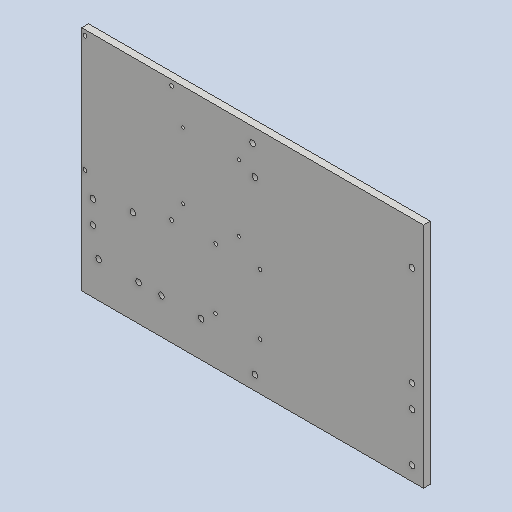
# Autodesk Inventor part: BackPlate
Saved by Autodesk Inventor 2023 (Build 270158000, 158)
## iProperties
Created: 2022-08-30
Part Number: BackPlate
Material: Generic
Document SubType Name: Modeling
Designer: Nathann
Density: 1 g/cm^3
Appearance: Default
Author: Nathann
Autodesk Inventor part; units mm, degrees
ref_plane "YZ Plane" through (0, 0, 0) normal (1, 0, 0) x (0, 1, 0)
ref_plane "XZ Plane" through (0, 0, 0) normal (0, 1, 0) x (-1, 0, 0)
ref_plane "XY Plane" through (0, 0, 0) normal (0, 0, 1) x (1, 0, 0)
sketch "Sketch1" plane through (0, 0, 0) normal (0, 1, 0) x (-1, 0, 0)
  line L0 (-150, -100) -> (150, -100)
  line L1 (150, -100) -> (150, 100)
  line L2 (150, 100) -> (-150, 100)
  line L3 (-150, 100) -> (-150, -100)
  line L4 (-150, -100) -> (150, 100) construction
  line L5 (150, -100) -> (-150, 100) construction
  point P0 (0, 0)
  dimension "d2" = 200
  dimension "d3" = 300
  constraints: 12 end point, 2 midpoint, 2 parallel, 1 horizontal, 1 perpendicular
  measures "d2" distance of L2.end L0.start
  measures "d3" distance of L0.start L0.end
extrude "Extrusion1" add sketch "Sketch1" along normal blind 6
sketch "Sketch2" plane through (0, 0, 0) normal (0, -1, 0) x (1, 0, 0)
  circle A0 centre (-11.9893, 68.6126) radius 1.35 projected
  circle A1 centre (-32.5352, -58.3765) radius 1.6 projected
  circle A2 centre (-32.4109, -5.3766) radius 1.6 projected
  circle A3 centre (6.589, -5.468) radius 1.6 projected
  circle A4 centre (-61.0635, 10.6754) radius 1.35 projected
  circle A5 centre (6.4647, -58.4679) radius 1.6 projected
  circle A6 centre (-12.0636, 10.6126) radius 1.35 projected
  circle A7 centre (-71.0314, 95.3283) radius 1.75 projected
  circle A8 centre (-147.0245, -6.6768) radius 1.75 projected
  circle A9 centre (-71.0245, -6.6717) radius 1.75 projected
  circle A10 centre (-147.0314, 95.3232) radius 1.75 projected
  circle A11 centre (-60.9892, 68.6754) radius 1.35 projected
  circle A12 centre (2.0404, -87.5) radius 2.5 projected
  circle A13 centre (140.0404, -87.5) radius 2.5 projected
  circle A14 centre (140.0404, 62.5) radius 2.5 projected
  circle A15 centre (2.0404, 62.5) radius 2.5 projected
  circle A16 centre (-100, -68.5) radius 2.5 projected
  circle A17 centre (-135, -68.5) radius 2.5 projected
  circle A18 centre (-80, -68.5) radius 2.5 projected
  circle A19 centre (-45, -68.5) radius 2.5 projected
  circle A20 centre (140.0262, -25) radius 2.5 projected
  circle A21 centre (140.0262, -45) radius 2.5 projected
  circle A22 centre (-139.9738, -25) radius 2.5 projected
  circle A23 centre (-139.9738, -45) radius 2.5 projected
  circle A24 centre (0.0123, 87.151) radius 2.5 projected
  circle A25 centre (-104.9877, -17.849) radius 2.5 projected
  point P0 (0, 0)
extrude "Extrusion2" cut sketch "Sketch2" against normal mid plane 30
equation "\"RodDiameter\" = 8"
equation "\"VerticalBearingOD\" = 16"
equation "\"PrintingClearance\" = 0.2"
equation "\"TubeID\" = 18"
equation "\"XLinearBearingOD\" = 19"
body "Solid1"
